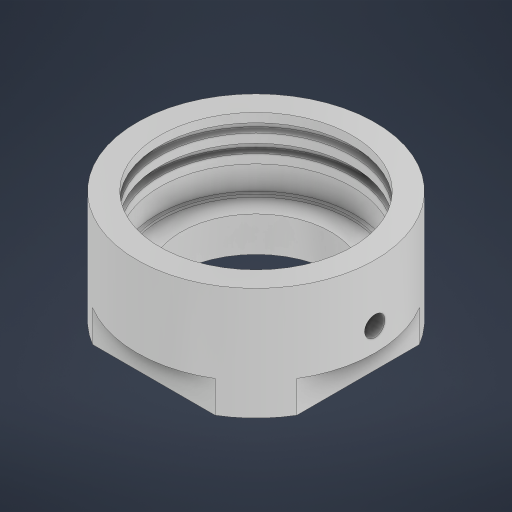
# Autodesk Inventor part: WashChamberConduit_1
Saved by Autodesk Inventor 2024 (Build 280153000, 153)
## iProperties
Created: 2025-02-18
Part Number: WashChamberConduit_1
Material: Aluminum 6061-AHC
Document SubType Name: Modeling
Designer: Tommy Rohmann
Density: 2.7 g/cm^3
Appearance: Aluminum - Dark
Author: Tommy Rohmann
Autodesk Inventor part; units mm, degrees
ref_plane "YZ Plane" through (0, 0, 0) normal (1, 0, 0) x (0, 1, 0)
ref_plane "XZ Plane" through (0, 0, 0) normal (0, 1, 0) x (-1, 0, 0)
ref_plane "XY Plane" through (0, 0, 0) normal (0, 0, 1) x (1, 0, 0)
sketch "WashChamberConduit" plane through (0, 0, 0) normal (0, 0, 1) x (1, 0, 0)
  line L0 (57.15, -1.8468) -> (59.3725, -1.8468)
  line L1 (57.15, -2.1643) -> (57.15, 31.7898)
  line L2 (57.785, 34.7292) -> (62.484, 34.7292)
  line L3 (62.484, 34.7292) -> (62.484, 29.3952)
  line L4 (62.484, 29.3952) -> (57.785, 29.3952)
  line L5 (57.785, 29.3952) -> (57.785, 24.0612)
  line L6 (57.785, 24.0612) -> (62.484, 24.0612)
  line L7 (62.484, 24.0612) -> (62.484, 18.7272)
  line L8 (59.3725, -1.8468) -> (59.3725, 13.3932)
  line L9 (57.785, 34.7292) -> (57.785, 40.0632)
  line L10 (57.785, 40.0632) -> (71.3867, 40.0632)
  line L11 (71.3867, -8.1968) -> (61.2267, -8.1968)
  line L12 (61.2267, -8.1968) -> (61.2267, -27.2468)
  line L13 (62.484, 18.7272) -> (57.785, 18.7272)
  line L14 (57.785, 18.7272) -> (57.785, 13.3932)
  line L15 (57.785, 13.3932) -> (59.3725, 13.3932)
  line L16 (0, -63.8087) -> (0, 25.5104)
  line L17 (71.3867, -8.1968) -> (71.3867, 40.0632)
  line L18 (57.15, -1.8468) -> (57.15, -3.4343)
  line L19 (61.2267, -27.2468) -> (71.3867, -27.2468)
  line L20 (71.3867, -27.2468) -> (71.3867, -8.1968)
  line L21 (59.3725, 5.7732) -> (71.3867, 5.7732)
  line L22 (57.15, -1.8468) -> (63.8852, -1.8468)
  line L23 (57.15, -3.4343) -> (44.8437, -3.4343)
  line L24 (44.8437, -3.4343) -> (48.8188, -27.2468)
  line L25 (61.2267, -27.2468) -> (48.8188, -27.2468)
  point P0 (52.07, -10.4939)
  dimension "d9" = 0.635
  dimension "d12" = 5.334
  dimension "d13" = 5.334
  dimension "d17" = 15.24
  dimension "d41" = 10.16
  dimension "d42" = 12.0142
  dimension "d44" = 114.3
  dimension "WashConduitOD" = 142.7734
  dimension "d46" = 1.5875
  dimension "d65" = 19.05
  dimension "d379" = 89.6874
  dimension "d381" = 25.4
  dimension "d382" = 97.6376
  dimension "d391" = 80.523
  dimension "d612" = 1.5875
  measures "d9" distance between parallel lines of L1 L9
  measures "d12" distance between parallel lines of L1 L3
  measures "d13" distance between parallel lines of L2 L10
  measures "d17" distance between parallel lines of L15 L0
  measures "d41" distance between parallel lines of L17 L12
  measures "d42" distance between parallel lines of L17 L8
  measures "d44" diameter of L1 L16
  measures "WashConduitOD" diameter of L17 L16
  measures "d46" distance of L0.start L18.end
  measures "d65" distance between parallel lines of L19 L11
  measures "d379" diameter of L23.end L16
  measures "d381" distance between parallel lines of L0 L25
  measures "d382" diameter of L24.end L16
  measures "d391" angle of L23 L24
  measures "d612" distance between parallel lines of L14 L8
derived "LAYOUT.ipt"
sketch "Sketch1" plane through (0, 0, 0) normal (0, 0, 1) x (1, 0, 0)
  line L0 (57.15, -1.8468) -> (59.3725, -1.8468)
  line L1 (57.15, -2.1643) -> (57.15, 31.7898)
  line L2 (57.785, 34.7292) -> (62.484, 34.7292)
  line L3 (62.484, 34.7292) -> (62.484, 29.3952)
  line L4 (62.484, 29.3952) -> (57.785, 29.3952)
  line L5 (57.785, 29.3952) -> (57.785, 24.0612)
  line L6 (57.785, 24.0612) -> (62.484, 24.0612)
  line L7 (62.484, 24.0612) -> (62.484, 18.7272)
  line L8 (59.3725, -1.8468) -> (59.3725, 13.3932)
  line L9 (57.785, 34.7292) -> (57.785, 40.0632)
  line L10 (57.785, 40.0632) -> (71.3867, 40.0632)
  line L11 (71.3867, -8.1968) -> (61.2267, -8.1968)
  line L12 (61.2267, -8.1968) -> (61.2267, -27.2468)
  line L13 (62.484, 18.7272) -> (57.785, 18.7272)
  line L14 (57.785, 18.7272) -> (57.785, 13.3932)
  line L15 (57.785, 13.3932) -> (59.3725, 13.3932)
  line L16 (0, -63.8087) -> (0, 25.5104)
  line L17 (71.3867, -8.1968) -> (71.3867, 40.0632)
  line L18 (57.15, -1.8468) -> (57.15, -3.4343)
  line L19 (61.2267, -27.2468) -> (71.3867, -27.2468)
  line L20 (71.3867, -27.2468) -> (71.3867, -8.1968)
  line L21 (59.3725, 5.7732) -> (71.3867, 5.7732)
  line L22 (57.15, -1.8468) -> (63.8852, -1.8468)
  line L23 (57.15, -3.4343) -> (44.8437, -3.4343)
  line L24 (44.8437, -3.4343) -> (48.8188, -27.2468)
  line L25 (61.2267, -27.2468) -> (48.8188, -27.2468)
revolve "Revolution1" add sketch "Sketch1" angle 90 mid plane about axis through (0, -63.8087, 0) along (0, 1, 0)
extrude "Extrusion1" cut sketch "Sketch1" along normal mid plane 254 contours L20 L19 L12 L11
ref_plane "Work Plane1" through (71.3867, 5.7732, 0) normal (1, 0, 0) x (0, 1, 0)
sketch "Sketch2" plane through (71.3867, 5.7732, 0) normal (1, 0, 0) x (0, 1, 0)
  circle A0 centre (0, 0) radius 6.0608
  point P0 (-5.7732, 0)
  constraints: 1 centre point
pattern_circular "Circular Pattern1" count 4 over 360 about axis through (0, -10, 0) along (0, 1, 0)
extrude "Extrusion2" cut sketch "Sketch2" along normal mid plane 68.2625
body "Solid1"
